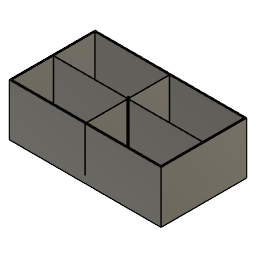
button (Autodesk Fusion 360 design; units mm, degrees)
part number: 2026-05-27-11-10-15-448
Autodesk Fusion 360 part; units mm, degrees
note: some values were not read from the file. Chosen so that the rebuilt part matches the saved one: which bodies a step acts on.
sketch "Sketch1" plane through (0, 0, 0) normal (0, 0, 1) x (1, 0, 0)
  line L0 (0, 0) -> (1, 0)
  line L1 (1, 0.2) -> (1, 0.7)
  line L2 (1, 0.9) -> (0, 0.9)
  line L3 (0, 0.2) -> (0, 0.7)
  line L4 (0.5, 0) -> (0.5, -30.05)
  line L5 (0.5, 0.9) -> (0.5, 30.95)
  line L6 (0, 0.45) -> (-53.5, 0.45)
  line L7 (1, 0.45) -> (54.5, 0.45)
  line L8 (54.5, 30.95) -> (-53.5, 30.95)
  line L9 (-53.5, 30.95) -> (-53.5, -30.05)
  line L10 (-53.5, -30.05) -> (54.5, -30.05)
  line L11 (54.5, -30.05) -> (54.5, 30.95)
  line L12 (-53.5, -30.05) -> (54.5, 30.95) construction
  line L13 (54.5, -30.05) -> (-53.5, 30.95) construction
  point P0 (0.3512, 0)
  point P1 (0.5, 0.45)
  point P2 (0.5, 0.9)
  point P3 (1, 0.45)
  point P4 (0.5, 0)
  point P5 (0, 0.45)
  dimension "d1" = 1
  dimension "d2" = 0.5
  dimension "d3" = 0.9
  dimension "d25" = 108
  dimension "d26" = 61
  constraint coincident L0.start origin
  constraint horizontal L0
  constraint vertical L1
  constraint perpendicular L1 L2
  constraint perpendicular L0 L3
  constraint coincident L0 P0
  constraint horizontal L8
  constraint vertical L9
  constraint horizontal L10
  constraint vertical L11
  constraint coincident L4.end L10
  constraint coincident L6.end L9
  constraint coincident L7.end L11
  constraint coincident L5.end L8
  constraint coincident P1 L12
  constraint coincident P1 L13
  constraint midpoint L2 P2
  constraint midpoint L1 P3
  constraint midpoint L0 P4
  constraint midpoint L3 P5
  constraint coincident P2 L5.start
  constraint perpendicular L2 L5
  constraint coincident P4 L4.start
  constraint coincident P3 L7.start
  constraint coincident P5 L6.start
  constraint perpendicular L3 L6
  measures "d1" distance of L0.start L0.end
  measures "d2" distance of L1.start L1.end
  measures "d3" distance of L0.end L2.start
  measures "d25" distance of L9.end L10.end
  measures "d26" distance of L8.end L9.end
extrude "Extrude1" add sketch "Sketch1" along normal blind 32 thin wall 0.1 centred open curves L7 L5 L6 L4 makes body 1 at (-17.8333, 0.4, 10.6667) makes body 2 at (18.8333, 0.5, 21.3333) makes body 3 at (0.45, 10.9167, 10.6667) makes body 4 at (0.55, -10.0167, 21.3333)
extrude "Extrude2" add sketch "Sketch1" along normal blind 32 thin wall 0.2 centred open curves L3 L1 bodies 1 2
extrude "Extrude3" add sketch "Sketch1" along normal blind 32 thin wall 0.3 centred open curves L2 L0 bodies 3 4
extrude "Extrude4" add sketch "Sketch1" against normal blind 5 bodies 1 2 3 4
extrude "Extrude5" add sketch "Sketch1" along normal blind 32 thin wall 1 on the right open curves L10 L11 L8 L9 bodies 1
sketch "Sketch2" plane through (0, 0, 32) normal (0, 0, 1) x (-1, 0, 0)
  line L0 (53.5, -30.95) -> (53.5, 30.05)
  line L1 (53.5, 30.05) -> (-0.45, 30.05)
  line L2 (-54.5, 30.05) -> (-54.5, -30.95)
  line L3 (-54.5, -30.95) -> (53.5, -30.95)
  line L4 (52.5, -0.5) -> (52.5, -29.95)
  line L5 (52.5, -29.95) -> (-0.45, -29.95)
  line L6 (-0.45, -29.95) -> (-0.45, -1.05)
  line L7 (-0.45, -1.05) -> (0, -1.05)
  line L8 (0, -1.05) -> (0, -0.75)
  line L9 (0, -0.75) -> (-1, -0.75)
  line L10 (-1, -0.75) -> (-1, -1.05)
  line L11 (-1, -1.05) -> (-0.55, -1.05)
  line L12 (-0.55, -1.05) -> (-0.55, -29.95)
  line L13 (-0.55, -29.95) -> (-53.5, -29.95)
  line L14 (-53.5, -29.95) -> (-53.5, -0.5)
  line L15 (-53.5, -0.5) -> (-1.1, -0.5)
  line L16 (-1.1, -0.5) -> (-1.1, -0.7)
  line L17 (-1.1, -0.7) -> (-0.9, -0.7)
  line L18 (-0.9, -0.7) -> (-0.9, -0.2)
  line L19 (-0.9, -0.2) -> (-1.1, -0.2)
  line L20 (-1.1, -0.2) -> (-1.1, -0.4)
  line L21 (-1.1, -0.4) -> (-53.5, -0.4)
  line L22 (-53.5, -0.4) -> (-53.5, 29.05)
  line L23 (-53.5, 29.05) -> (-0.55, 29.05)
  line L24 (-0.55, 29.05) -> (-0.55, 0.15)
  line L25 (-0.55, 0.15) -> (-1, 0.15)
  line L26 (-1, 0.15) -> (-1, -0.15)
  line L27 (-1, -0.15) -> (0, -0.15)
  line L28 (0, -0.15) -> (0, 0.15)
  line L29 (0, 0.15) -> (-0.45, 0.15)
  line L30 (-0.45, 0.15) -> (-0.45, 29.05)
  line L31 (-0.45, 29.05) -> (52.5, 29.05)
  line L32 (52.5, 29.05) -> (52.5, -0.4)
  line L33 (52.5, -0.4) -> (0.1, -0.4)
  line L34 (0.1, -0.4) -> (0.1, -0.2)
  line L35 (0.1, -0.2) -> (-0.1, -0.2)
  line L36 (-0.1, -0.2) -> (-0.1, -0.7)
  line L37 (-0.1, -0.7) -> (0.1, -0.7)
  line L38 (0.1, -0.7) -> (0.1, -0.5)
  line L39 (0.1, -0.5) -> (52.5, -0.5)
  line L40 (0, -0.1704) -> (-1, -0.1704)
  line L41 (-1, -0.1704) -> (-1, 0.15)
  line L42 (-1, 0.15) -> (0, 0.15)
  line L43 (0, 0.15) -> (0, -0.1704)
  line L44 (0, -0.728) -> (-1, -0.728)
  line L45 (-1, -0.728) -> (-1, -1.05)
  line L46 (-1, -1.05) -> (0, -1.05)
  line L47 (0, -1.05) -> (0, -0.728)
  line L48 (-0.45, 30.05) -> (-0.55, 30.05)
  line L49 (-0.55, 30.05) -> (-54.5, 30.05)
  constraint horizontal L40
  constraint vertical L41
  constraint horizontal L42
  constraint vertical L43
  constraint coincident L25.end L26.start
  constraint horizontal L44
  constraint vertical L45
  constraint horizontal L46
  constraint vertical L47
  constraint coincident L10.end L11.start
extrude "Extrude6" add sketch "Sketch2" along normal blind 1 contours L7 L8 L9 L10 L11 L45 L46 L47 | L9 L44 L45 L47 | L25 L26 L27 L28 L29 L41 L42 L43 | L27 L40 L41 L43 bodies 1
